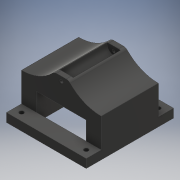
# Autodesk Inventor part: Sujetador para corte superior
Saved by Autodesk Inventor 2018 (Build 220112000, 112)
## iProperties
Created: 2019-05-21
Part Number: Sujetador para corte superior
Material: Generic
Document SubType Name: Modeling
Designer: Iván
Density: 1 g/cm^3
Appearance: Default
Author: Iván
Autodesk Inventor part; units mm, degrees
ref_plane "YZ Plane" through (0, 0, 0) normal (1, 0, 0) x (0, 1, 0)
ref_plane "XZ Plane" through (0, 0, 0) normal (0, 1, 0) x (-1, 0, 0)
ref_plane "XY Plane" through (0, 0, 0) normal (0, 0, 1) x (1, 0, 0)
sketch "Sketch1" plane through (0, 0, 0) normal (0, 0, 1) x (1, 0, 0)
  line L0 (-37, 40.5) -> (37, 40.5)
  line L1 (37, 40.5) -> (37, -40.5)
  line L2 (37, -40.5) -> (-37, -40.5)
  line L3 (-37, -40.5) -> (-37, 40.5)
  line L4 (-30, 33.5) -> (30, 33.5) construction
  line L5 (30, 33.5) -> (30, -33.5) construction
  line L6 (30, -33.5) -> (-30, -33.5) construction
  line L7 (-30, -33.5) -> (-30, 33.5) construction
  line L8 (23, 26.5) -> (-23, 26.5)
  line L9 (-23, 26.5) -> (-23, -26.5)
  line L10 (-23, -26.5) -> (23, -26.5)
  line L11 (23, -26.5) -> (23, 26.5)
  point P0 (0, 0)
  point P1 (0, 40.5)
  point P2 (-37, 0)
  point P3 (0, 33.5)
  point P4 (30, 0)
  dimension "d0" = 81
  dimension "d1" = 74
  dimension "d2" = 7
  dimension "d3" = 7
  dimension "d4" = 14
  constraints: 24 end point, 6 parallel, 4 coincident, 4 midpoint, 3 perpendicular, 2 horizontal, 2 horizontal alignment, 2 vertical alignment, 3 other
  measures "d0" distance of L0.end L1.end
  measures "d1" distance between parallel lines of L1 L3
  measures "d2" distance between parallel lines of L0 L4
  measures "d3" distance between parallel lines of L3 L7
  measures "d4" distance between parallel lines of L0 L8
extrude "Extrusion1" add sketch "Sketch1" along normal blind 8
hole "Hole1" at (-30, 33.5, 0) at (30, 33.5, 0) at (30, -33.5, 0) at (-30, -33.5, 0) direction (0, 0, 1) diameter 4 end through all
sketch "Sketch2" plane through (0, 0, 8) normal (0, 0, 1) x (1, 0, 0)
  line L0 (0, 0) -> (0, 37) construction
  line L1 (-23, 26.5) -> (-37, 26.5)
  line L2 (-37, 26.5) -> (-37, -26.5)
  line L3 (-37, -26.5) -> (-23, -26.5)
  line L4 (-23, -26.5) -> (-23, 26.5)
  line L5 (-23, 26.5) -> (23, 26.5) projected
  line L6 (-23, -26.5) -> (-23, 26.5) projected
  line L7 (-37, 40.5) -> (-37, -40.5) projected
  line L8 (23, -26.5) -> (-23, -26.5) projected
  line L9 (23, 26.5) -> (37, 26.5)
  line L10 (37, 26.5) -> (37, -26.5)
  line L11 (37, -26.5) -> (23, -26.5)
  line L12 (23, -26.5) -> (23, 26.5)
  line L13 (23, 26.5) -> (23, -26.5) projected
  line L14 (37, -40.5) -> (37, 40.5) projected
  constraints: 18 end point, 8 collinear, 4 parallel, 2 horizontal, 2 perpendicular, 1 vertical
extrude "Extrusion2" add sketch "Sketch2" along normal blind 27 contours L4 L3 L2 L1 | L9 L10 L11 L12
sketch "Sketch3" plane through (-23, -26.5, 0) normal (1, 0, 0) x (0, 0, -1)
  line L0 (-35, 0) -> (-25, 0)
  line L1 (-25, 0) -> (-25, 53)
  line L2 (-25, 53) -> (-35, 53)
  line L3 (-35, 53) -> (-35, 0)
  line L4 (-8, 53) -> (-35, 53) projected
  line L5 (-35, 0) -> (-35, 53) projected
  line L6 (-8, 0) -> (-35, 0) projected
  point P0 (0, 26.5)
  dimension "d16" = 10
  constraints: 8 end point, 3 collinear, 2 parallel, 1 horizontal, 1 perpendicular
  measures "d16" distance between parallel lines of L1 L3
extrude "Extrusion3" add sketch "Sketch3" along normal up to next
sketch "Sketch4" plane through (0, 0, 35) normal (0, 0, 1) x (1, 0, 0)
  line L0 (-9.525, 26.5) -> (9.525, 26.5)
  line L1 (9.525, 26.5) -> (9.525, -26.5)
  line L2 (9.525, -26.5) -> (-9.525, -26.5)
  line L3 (-9.525, -26.5) -> (-9.525, 26.5)
  line L4 (37, 26.5) -> (-37, 26.5) projected
  point P0 (0, 0)
  point P1 (9.525, 0)
  point P2 (0, 26.5)
  dimension "d19" = 19.05
  constraints: 8 end point, 2 midpoint, 2 parallel, 1 collinear, 1 horizontal, 1 horizontal alignment, 1 perpendicular, 1 vertical alignment
  measures "d19" distance between parallel lines of L3 L1
extrude "Extrusion4" add sketch "Sketch4" along normal blind 13.7
ref_plane "Work Plane1" through (-37, -22, 8) normal (0, -1, 0) x (1, 0, 0)
sketch "Sketch5" plane through (-37, -22, 8) normal (0, -1, 0) x (1, 0, 0)
  line L0 (27.475, 40.7) -> (46.525, 40.7) projected
  circle A0 centre (37, 39.7) radius 6.35
  point P0 (37, -8)
  point P1 (37, 40.7)
  dimension "d23" = 12.7
  dimension "d24" = 1
  constraints: 1 centre point, 1 midpoint, 1 vertical alignment
  measures "d23" diameter of A0
  measures "d24" distance from line of L0 A0.centre
hole "Hole2" at (0, -22, 47.7) direction (0, 1, 0) diameter 12.7 depth 44
sketch "Sketch6" plane through (-37, -26.5, 8) normal (0, -1, 0) x (1, 0, 0)
  circle A0 centre (37, 39.7) radius 6.35 projected
  circle A1 centre (37, 36.525) radius 1.5
  point P0 (37, -8)
  dimension "d32" = 3
  dimension "d33" = 3.175
  constraints: 1 centre point, 1 vertical alignment
  measures "d32" diameter of A1
  measures "d33" distance of A0.centre A1.centre
hole "Hole3" at (0, -26.5, 44.525) direction (0, 1, 0) diameter 3 end through all
fillet "Fillet1" radius 5 2 edges at (9.525, 0, 48.7) (-9.525, 0, 48.7)
fillet "Fillet2" radius 40 2 edges at (9.525, 0, 35) (-9.525, 0, 35)
equation "\"d4\" = 2 * d2"
body "Solid1"
